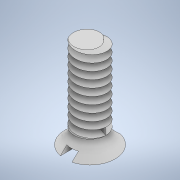
# Autodesk Inventor part: Винт 3x12
Saved by Autodesk Inventor 2020 (Build 240168000, 168)
## iProperties
Created: 2021-04-26
Part Number: Винт 3x12
Material: Типовые
Document SubType Name: Modeling
Designer: lbfas
Density: 1 g/cm^3
Appearance: По умолчанию
Author: lbfas
Autodesk Inventor part; units mm, degrees
ref_plane "YZ Plane" through (0, 0, 0) normal (1, 0, 0) x (0, 1, 0)
ref_plane "XY Plane" through (0, 0, 0) normal (0, 0, 1) x (1, 0, 0)
sketch "Эскиз1" plane through (0, 0, 0) normal (0, 1, 0) x (-1, 0, 0)
  circle A0 centre (0, 0) radius 4
  dimension "d0" = 8
  constraints: 1 centre point, 1 coincident
  measures "d0" diameter of A0
ref_plane "РабПлоскость1" through (0, 2.5, 0) normal (0, 1, 0) x (-1, 0, 0)
sketch "Эскиз2" plane through (0, 2.5, 0) normal (0, 1, 0) x (-1, 0, 0)
  circle A0 centre (0, 0) radius 1.5
  dimension "d2" = 3
  constraints: 1 centre point, 1 coincident
  measures "d2" diameter of A0
loft "Лофт1" add profiles "Эскиз1", "Эскиз2"
sketch "Эскиз3" plane through (0, 2.5, 0) normal (0, 1, 0) x (1, 0, 0)
  circle A0 centre (0, 0) radius 2.5
  constraints: 1 centre point, 1 coincident
extrude "Выдавливание1" add sketch "Эскиз3" along normal blind 12
sketch "Эскиз4" plane through (0, 0, 0) normal (0, 0, 1) x (1, 0, 0)
  line L0 (2.5, 3.0774) -> (1.5, 3.0774)
  line L1 (1.5, 3.0774) -> (2.5, 2.5)
  line L2 (2.5, 3.0774) -> (2.5, 2.5)
  line L3 (1.5, 3.0774) -> (2.5, 3.6547)
  line L4 (2.5, 3.0774) -> (2.5, 3.6547)
  line L5 (2.5, 14.5) -> (-2.5, 14.5) projected
  line L6 (2.5, 2.5) -> (-2.5, 2.5) projected
  line L7 (2.5, 2.5) -> (1.9783, 2.5)
  point P0 (0, 0)
  dimension "d10" = 30
  constraints: 12 end point, 1 perpendicular, 1 point on line
  measures "d10" angle of L1 L0
coil "Пружина1" sketch "Эскиз4" operation cut axis through (0, 2.5, 0) along (0, 1, 0) pitch 1.155 turns 10.822511 hand left
sketch "Эскиз5" plane through (0, 0, 0) normal (0, -1, 0) x (1, 0, 0)
  line L0 (-0.8, 0.9798) -> (-0.8, -3.9192)
  circle A0 centre (0, 0) radius 4 projected
  line L1 (-0.8, 0.9798) -> (-0.8, 5.8788)
  line L2 (1, 0) -> (1, -4.899)
  line L3 (1, 0) -> (1, 4.899)
  point P0 (1, 3.873)
  point P1 (-0.8, 3.9192)
  point P2 (1, -3.873)
  constraints: 8 end point, 2 other
extrude "Выдавливание2" cut sketch "Эскиз5" against normal blind 1 contours L1 A0 L3 L2 L0
